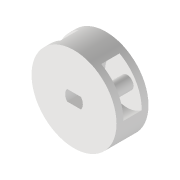
# Autodesk Inventor part: Pump_Rotatio_new.
Saved by Autodesk Inventor 2022.5 (Build 265521000, 521)
## iProperties
Created: 2022-11-30
Part Number: Pump_Rotatio_new.
Material: Generisch
Document SubType Name: Modeling
Designer: diederichbenedict
Density: 1 g/cm^3
Appearance: Vorgabe
Author: diederichbenedict
Autodesk Inventor part; units mm, degrees
ref_plane "YZ Plane" through (0, 0, 0) normal (1, 0, 0) x (0, 1, 0)
ref_plane "XZ Plane" through (0, 0, 0) normal (0, 1, 0) x (-1, 0, 0)
ref_plane "XY Plane" through (0, 0, 0) normal (0, 0, 1) x (1, 0, 0)
sketch "Skizze3" plane through (0, 0, 0) normal (0, 0, 1) x (1, 0, 0)
  circle A0 centre (82.7359, -97.3647) radius 1.5 projected
  circle A1 centre (87.3441, -89.6424) radius 2.7776 projected
  circle A2 centre (0, 0) radius 12.5
  line L0 (0, -9.5) -> (-8.2272, 4.75)
  line L1 (-8.2272, 4.75) -> (8.2272, 4.75)
  line L2 (8.2272, 4.75) -> (0, -9.5)
  circle A3 centre (0, -9.5) radius 1.9
  circle A4 centre (8.2272, 4.75) radius 1.9
  circle A5 centre (-8.2272, 4.75) radius 1.9
  circle A6 centre (0, 0) radius 2.6
  line L3 (-2.0494, -1.6) -> (2.0494, -1.6)
  line L4 (-2.0494, 1.6) -> (2.0494, 1.6)
  circle A7 centre (8.2272, 4.75) radius 2 construction
  dimension "d10" = 25
  dimension "d11" = 9.5
  dimension "d12" = 3.8
  dimension "d13" = 3.8
  dimension "d14" = 3.8
  dimension "d15" = 5.2
  dimension "d16" = 1.6
  dimension "d17" = 1.6
  constraints: 10 end point, 6 coincident, 5 centre point, 4 point on circle, 1 horizontal, 7 other
  measures "d10" diameter of A2
  measures "d11" distance of L0.start point (0, 0)
  measures "d12" diameter of A3
  measures "d13" diameter of A4
  measures "d14" diameter of A5
  measures "d15" diameter of A6
  measures "d16" distance from line of point (0, 0) L3
  measures "d17" distance from line of L4 A2.centre
extrude "Extrusion3" add sketch "Skizze3" along normal blind 2 contours A2 | L0 A5 L1 A4 L2 A3 | L4 A6 | A6 L3
sketch "Skizze4" plane through (0, 0, 0) normal (0, 0, -1) x (-1, 0, 0)
  circle A0 centre (0, 0) radius 12.5 projected
  circle A1 centre (8.2272, 4.75) radius 1.9 projected
  circle A2 centre (0, -9.5) radius 1.9 projected
  arc A3 (-2.0494, 1.6) -> (-2.0494, -1.6) centre (0, 0) ccw projected
  line L0 (2.0494, 1.6) -> (-2.0494, 1.6) projected
  arc A4 (2.0494, -1.6) -> (2.0494, 1.6) centre (0, 0) ccw projected
  line L1 (-2.0494, -1.6) -> (2.0494, -1.6) projected
  circle A5 centre (-8.2272, 4.75) radius 1.9 projected
  circle A6 centre (0, -9.5) radius 6.5
  circle A7 centre (-8.2272, 4.75) radius 6.5
  circle A8 centre (8.2272, 4.75) radius 6.5
  line L2 (-6.5, -16) -> (6.4807, -16)
  line L3 (6.4807, -16) -> (6.4807, -9)
  line L4 (6.4807, -9) -> (-6.5, -9)
  line L5 (-6.5, -9) -> (-6.5, -16)
  line L6 (-6.5, -16) -> (6.4807, -9) construction
  line L7 (6.4807, -16) -> (-6.5, -9) construction
  line L8 (5.8481, -4.1292) -> (17.1064, 2.3708)
  line L9 (17.1064, 2.3708) -> (10.6064, 13.6292)
  line L10 (10.6064, 13.6292) -> (-0.6519, 7.1292)
  line L11 (-0.6519, 7.1292) -> (5.8481, -4.1292)
  line L12 (5.8481, -4.1292) -> (10.6064, 13.6292) construction
  line L13 (17.1064, 2.3708) -> (-0.6519, 7.1292) construction
  line L14 (0, 0) -> (8.2272, 4.75)
  line L15 (8.2272, 4.75) -> (0, 0)
  line L16 (0, 0) -> (-8.4804, 4.8962)
  line L17 (-5.8481, -4.1292) -> (0.6519, 7.1292)
  line L18 (0.6519, 7.1292) -> (-11.1127, 13.9215)
  line L19 (-11.1127, 13.9215) -> (-17.6127, 2.6631)
  line L20 (-17.6127, 2.6631) -> (-5.8481, -4.1292)
  line L21 (-5.8481, -4.1292) -> (-11.1127, 13.9215) construction
  line L22 (0.6519, 7.1292) -> (-17.6127, 2.6631) construction
  point P0 (6.1204, 10.8991)
  point P1 (12.4991, -0.1491)
  point P2 (-6.1204, 10.8991)
  point P3 (-12.4991, -0.1491)
  point P4 (-6.3787, -10.75)
  point P5 (6.3787, -10.75)
  point P6 (-0.0096, -12.5)
  point P7 (-11.4772, -0.8792)
  point P8 (-12.4966, -0.2906)
  point P9 (-6.5, -10.6771)
  point P10 (-6.5, -9.5)
  point P11 (6.4807, -10.6888)
  point P12 (12.4966, -0.2906)
  point P13 (11.4772, -0.8792)
  point P14 (4.9772, 10.3792)
  point P15 (5.9966, 10.9677)
  point P16 (-5.9966, 10.9677)
  point P17 (-4.9772, 10.3792)
  dimension "d20" = 13
  dimension "d21" = 13
  dimension "d22" = 13
  constraints: 42 end point, 7 parallel, 6 midpoint, 5 tangent, 4 perpendicular, 3 coincident, 2 centre point, 2 horizontal, 1 collinear, 1 vertical, 5 other
  measures "d21" diameter of A7
  measures "d22" diameter of A8
extrude "Extrusion4" add sketch "Skizze4" along normal blind 2.7 contours L10 L18 A0 | A8 L11 L17 L18 L10 | A0 L3 A6 L4 L5 L20 L17 L16 A3 L1 A4 L14 L11 L8 | L8 L11 A8 | L14 A4 L0 A3 L16 L17 L11 | L18 L17 L11 L10 | L10 L11 L17 A7 L18 | L3 A6 | L17 L20 A7 | L5 L4 A6
sketch "Skizze9" plane through (0, 0, 0) normal (0, 0, -1) x (-1, 0, 0)
  circle A0 centre (-8.2272, 4.75) radius 1.9 projected
  circle A1 centre (8.2272, 4.75) radius 1.9 projected
  circle A2 centre (0, -9.5) radius 1.9 projected
  point P0 (0, 0)
extrude "Extrusion7" add sketch "Skizze9" along normal blind 2.7 and the other way blind 2
mirror "Spiegeln1" about plane through (0, 0.9056, -2.7) normal (0, 0, -1) of "Extrusion3", "Extrusion4", "Extrusion7"
equation "\"d12\" = d13"
equation "\"d14\" = d13"
equation "\"d17\" = d16"
equation "\"d20\" = d21"
equation "\"d22\" = d21"
